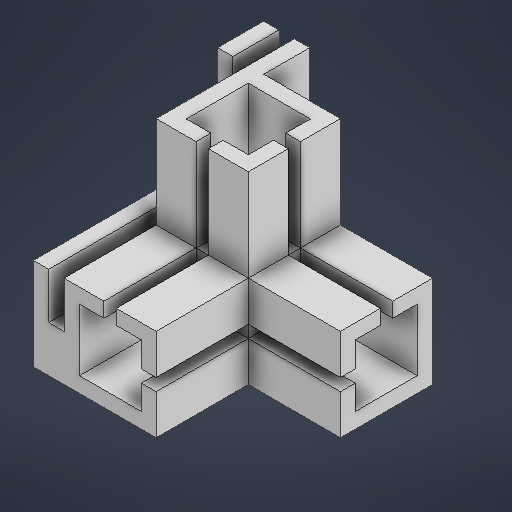
# Autodesk Inventor part: corner connector with rails (front right)
Saved by Autodesk Inventor 2026.2 (Build 302298000, 298)
## iProperties
Created: 2025-11-17
Part Number: corner connector with rails (front right)
Material: Generic
Document SubType Name: Modeling
Designer: dongr
Density: 1 g/cm^3
Appearance: Default
Author: dongr
Autodesk Inventor part; units mm, degrees
ref_plane "YZ Plane" through (0, 0, 0) normal (1, 0, 0) x (0, 1, 0)
ref_plane "XZ Plane" through (0, 0, 0) normal (0, 1, 0) x (-1, 0, 0)
ref_plane "XY Plane" through (0, 0, 0) normal (0, 0, 1) x (1, 0, 0)
sketch "Sketch1" plane through (0, 0, 0) normal (0, 0, 1) x (1, 0, 0)
  line L0 (0, 0) -> (38.1, 0)
  line L1 (38.1, 0) -> (38.1, 38.1)
  line L2 (38.1, 38.1) -> (0, 38.1)
  line L3 (0, 38.1) -> (0, 0)
  dimension "d0" = 38.1
  dimension "d1" = 38.1
  constraints: 8 end point, 2 parallel, 1 horizontal, 1 perpendicular
  measures "d0" distance of L2.end L1.end
  measures "d1" distance of L1.end L0.end
extrude "Extrusion1" add sketch "Sketch1" along normal blind 38.1
sketch "Sketch2" plane through (0, 0, 38.1) normal (0, 0, 1) x (1, 0, 0)
  line L0 (6.35, 6.35) -> (32.004, 6.35)
  line L1 (32.004, 6.35) -> (32.004, 32.004)
  line L2 (32.004, 32.004) -> (6.35, 32.004)
  line L3 (6.35, 32.004) -> (6.35, 6.35)
  line L4 (38.1, 0) -> (38.1, 38.1) projected
  line L5 (0, 0) -> (38.1, 0)
  line L6 (38.1, 0) -> (38.1, 38.1)
  line L7 (38.1, 38.1) -> (0, 38.1)
  line L8 (0, 38.1) -> (0, 0)
  dimension "d4" = 25.654
  dimension "d5" = 25.654
  constraints: 16 end point, 4 parallel, 2 horizontal, 2 perpendicular
  measures "d4" distance of L2.end L1.end
  measures "d5" distance of L1.end L0.end
extrude "Extrusion2" cut sketch "Sketch2" against normal blind 31.75 contours L3 L2 L1 L0
sketch "Sketch5" plane through (0, 0, 38.1) normal (0, 0, 1) x (1, 0, 0)
  line L0 (6.35, 6.35) -> (6.35, 32.004) projected
  line L1 (6.35, 6.35) -> (32.004, 6.35)
  line L2 (32.004, 6.35) -> (32.004, 32.004)
  line L3 (32.004, 32.004) -> (6.35, 32.004)
  line L4 (6.35, 32.004) -> (6.35, 6.35)
  line L5 (0, 0) -> (38.1, 0) projected
  line L6 (0, 0) -> (38.1, 0)
  line L7 (38.1, 0) -> (38.1, 38.1)
  line L8 (38.1, 38.1) -> (0, 38.1)
  line L9 (0, 38.1) -> (0, 0)
  constraints: 16 end point, 4 parallel, 2 horizontal, 2 perpendicular
extrude "Extrusion4" add sketch "Sketch5" along normal blind 38.1
sketch "Sketch7" plane through (38.1, 0, 0) normal (1, 0, 0) x (0, 0, -1)
  line L0 (0, 0) -> (-76.2, 0) projected
  line L1 (0, 0) -> (-38.1, 0)
  line L2 (-38.1, 0) -> (-38.1, 38.1)
  line L3 (-38.1, 38.1) -> (0, 38.1)
  line L4 (0, 38.1) -> (0, 0)
  line L5 (-76.2, 6.35) -> (-6.35, 6.35) projected
  line L6 (-6.35, 6.35) -> (-32.004, 6.35)
  line L7 (-32.004, 6.35) -> (-32.004, 32.004)
  line L8 (-32.004, 32.004) -> (-6.35, 32.004)
  line L9 (-6.35, 32.004) -> (-6.35, 6.35)
  dimension "d16" = 38.1
  dimension "d17" = 38.1
  dimension "d20" = 25.654
  dimension "d21" = 25.654
  constraints: 16 end point, 4 parallel, 2 horizontal, 2 perpendicular
  measures "d16" distance of L2.end L3.end
  measures "d17" distance of L1.end L2.end
  measures "d20" distance of L7.end L8.end
  measures "d21" distance of L6.end L7.end
extrude "Extrusion6" add sketch "Sketch7" along normal blind 38.1
sketch "Sketch9" plane through (38.1, 6.35, 6.35) normal (1, 0, 0) x (0, 0, -1)
  line L0 (-25.654, 0) -> (-25.654, 25.654) projected
  line L1 (0, 0) -> (0, 25.654) projected
  line L2 (-25.654, 0) -> (0, 0)
  line L3 (0, 0) -> (0, 25.654)
  line L4 (0, 25.654) -> (-25.654, 25.654)
  line L5 (-25.654, 25.654) -> (-25.654, 0)
  point P0 (6.35, -6.35)
  constraints: 8 end point, 2 parallel, 1 horizontal, 1 perpendicular
extrude "Extrusion7" cut sketch "Sketch9" against normal blind 31.75
sketch "Sketch10" plane through (0, 38.1, 76.2) normal (0, 1, 0) x (1, 0, 0)
  line L0 (76.2, 69.85) -> (6.35, 69.85) projected
  line L1 (6.35, 69.85) -> (32.004, 69.85)
  line L2 (32.004, 69.85) -> (32.004, 44.196)
  line L3 (32.004, 44.196) -> (6.35, 44.196)
  line L4 (6.35, 44.196) -> (6.35, 69.85)
  line L5 (38.1, 38.1) -> (38.1, 0) projected
  line L6 (0, 76.2) -> (0, 0) projected
  line L7 (38.1, 38.1) -> (0, 38.1)
  line L8 (0, 38.1) -> (0, 76.2)
  line L9 (0, 76.2) -> (38.1, 76.2)
  line L10 (38.1, 76.2) -> (38.1, 38.1)
  point P0 (0, 38.1)
  dimension "d26" = 25.654
  dimension "d27" = 25.654
  constraints: 16 end point, 4 parallel, 2 horizontal, 2 perpendicular
  measures "d26" distance of L2.end L3.end
  measures "d27" distance of L1.end L2.end
extrude "Extrusion8" add sketch "Sketch10" along normal blind 38.1
sketch "Sketch11" plane through (6.35, 38.1, 6.35) normal (0, 1, 0) x (1, 0, 0)
  line L0 (0, -25.654) -> (25.654, -25.654) projected
  line L1 (25.654, -25.654) -> (0, -25.654)
  line L2 (0, -25.654) -> (0, 0)
  line L3 (0, 0) -> (25.654, 0)
  line L4 (25.654, 0) -> (25.654, -25.654)
  point P0 (-6.35, 6.35)
  constraints: 8 end point, 2 parallel, 1 horizontal, 1 perpendicular
extrude "Extrusion9" cut sketch "Sketch11" against normal blind 6.35
sketch "Sketch12" plane through (0, 76.2, 76.2) normal (0, 1, 0) x (1, 0, 0)
  line L0 (38.1, 55.88) -> (32.004, 55.88)
  line L1 (32.004, 55.88) -> (32.004, 58.42)
  line L2 (32.004, 58.42) -> (38.1, 58.42)
  line L3 (38.1, 58.42) -> (38.1, 55.88)
  point P0 (0, 76.2)
  dimension "d32" = 6.096
  dimension "d33" = 2.54
  constraints: 8 end point, 2 parallel, 1 horizontal, 1 perpendicular
  measures "d32" distance of L1.end L2.end
  measures "d33" distance of L0.end L1.end
extrude "Extrusion10" cut sketch "Sketch12" against normal blind 38.1
sketch "Sketch13" plane through (76.2, 38.1, 38.1) normal (0, 1, 0) x (1, 0, 0)
  line L0 (0, 31.75) -> (0, 6.096) projected
  line L1 (-44.196, 17.78) -> (0, 17.78)
  line L2 (0, 17.78) -> (0, 20.32)
  line L3 (0, 20.32) -> (-44.196, 20.32)
  line L4 (-44.196, 20.32) -> (-44.196, 17.78)
  point P0 (-76.2, 38.1)
  dimension "d36" = 2.54
  constraints: 8 end point, 2 parallel, 1 horizontal, 1 perpendicular, 1 point on line
  measures "d36" distance of L2.end L1.end
extrude "Extrusion11" cut sketch "Sketch13" against normal blind 6.35
sketch "Sketch15" plane through (0, 76.2, 76.2) normal (0, 1, 0) x (1, 0, 0)
  line L0 (17.78, 38.1) -> (20.32, 38.1)
  line L1 (20.32, 38.1) -> (20.32, 44.196)
  line L2 (20.32, 44.196) -> (17.78, 44.196)
  line L3 (17.78, 44.196) -> (17.78, 38.1)
  point P0 (0, 76.2)
  dimension "d39" = 2.54
  dimension "d40" = 6.096
  constraints: 8 end point, 2 parallel, 1 horizontal, 1 perpendicular
  measures "d39" distance of L2.end L1.end
  measures "d40" distance of L1.end L0.end
extrude "Extrusion12" cut sketch "Sketch15" against normal blind 38.1
sketch "Sketch16" plane through (0, 38.1, 76.2) normal (0, 1, 0) x (1, 0, 0)
  line L0 (20.32, 44.196) -> (20.32, 38.1) projected
  line L1 (0, 0) -> (38.1, 0) projected
  line L2 (20.32, 44.196) -> (17.78, 44.196)
  line L3 (17.78, 44.196) -> (17.78, 0)
  line L4 (17.78, 0) -> (20.32, 0)
  line L5 (20.32, 0) -> (20.32, 44.196)
  point P0 (0, 76.2)
  dimension "d43" = 2.54
  constraints: 8 end point, 2 parallel, 1 horizontal, 1 perpendicular, 1 point on line
  measures "d43" distance of L4.end L3.end
extrude "Extrusion13" cut sketch "Sketch16" against normal blind 6.35
sketch "Sketch17" plane through (38.1, 0, 76.2) normal (1, 0, 0) x (0, 0, -1)
  line L0 (38.1, 0) -> (38.1, 38.1) projected
  line L1 (0, 17.78) -> (38.1, 17.78)
  line L2 (38.1, 17.78) -> (38.1, 20.32)
  line L3 (38.1, 20.32) -> (0, 20.32)
  line L4 (0, 20.32) -> (0, 17.78)
  point P0 (76.2, 0)
  dimension "d46" = 2.54
  constraints: 8 end point, 2 parallel, 1 horizontal, 1 perpendicular, 1 point on line
  measures "d46" distance of L2.end L1.end
extrude "Extrusion14" cut sketch "Sketch17" against normal blind 6.35
sketch "Sketch18" plane through (38.1, 0, 38.1) normal (0, 0, 1) x (1, 0, 0)
  line L0 (0, 17.78) -> (38.1, 17.78)
  line L1 (38.1, 17.78) -> (38.1, 20.32)
  line L2 (38.1, 20.32) -> (0, 20.32)
  line L3 (0, 20.32) -> (0, 17.78)
  point P0 (-38.1, 0)
  dimension "d49" = 38.1
  dimension "d50" = 2.54
  constraints: 8 end point, 2 parallel, 1 horizontal, 1 perpendicular
  measures "d49" distance of L2.end L1.end
  measures "d50" distance of L1.end L0.end
extrude "Extrusion15" cut sketch "Sketch18" against normal blind 6.35
sketch "Sketch20" plane through (38.1, 38.1, 38.1) normal (0, 0, 1) x (1, 0, 0)
  line L0 (-17.78, -6.096) -> (-17.78, 38.1) projected
  line L1 (0, 0) -> (-17.78, 0) projected
  line L2 (-17.78, 38.1) -> (-16.51, 38.1)
  line L3 (-16.51, 38.1) -> (-16.51, 0)
  line L4 (-16.51, 0) -> (-17.78, 0)
  line L5 (-17.78, 0) -> (-17.78, 38.1)
  point P0 (-38.1, -38.1)
  dimension "d53" = 1.27
  constraints: 8 end point, 2 parallel, 1 horizontal, 1 perpendicular, 1 point on line
  measures "d53" distance of L3.end L4.end
extrude "Extrusion16" cut sketch "Sketch20" against normal blind 6.35
sketch "Sketch21" plane through (38.1, 38.1, 76.2) normal (0, 1, 0) x (1, 0, 0)
  line L0 (-17.78, 0) -> (-17.78, 44.196) projected
  line L1 (0, 0) -> (-17.78, 0) projected
  line L2 (-17.78, 44.196) -> (-16.51, 44.196)
  line L3 (-16.51, 44.196) -> (-16.51, 0)
  line L4 (-16.51, 0) -> (-17.78, 0)
  line L5 (-17.78, 0) -> (-17.78, 44.196)
  point P0 (-38.1, 76.2)
  dimension "d56" = 1.27
  constraints: 8 end point, 2 parallel, 1 horizontal, 1 perpendicular, 1 point on line
  measures "d56" distance of L3.end L4.end
extrude "Extrusion17" cut sketch "Sketch21" against normal blind 6.35
sketch "Sketch23" plane through (0, 38.1, 38.1) normal (0, 0, 1) x (1, 0, 0)
  line L0 (17.78, 0) -> (17.78, 38.1) projected
  line L1 (17.78, 0) -> (0, 0) projected
  line L2 (17.78, 38.1) -> (16.51, 38.1)
  line L3 (16.51, 38.1) -> (16.51, 0)
  line L4 (16.51, 0) -> (17.78, 0)
  line L5 (17.78, 0) -> (17.78, 38.1)
  point P0 (0, -38.1)
  dimension "d59" = 1.27
  constraints: 8 end point, 2 parallel, 1 horizontal, 1 perpendicular, 1 point on line
  measures "d59" distance of L4.end L3.end
extrude "Extrusion18" cut sketch "Sketch23" against normal blind 6.35
sketch "Sketch24" plane through (0, 38.1, 76.2) normal (0, 1, 0) x (1, 0, 0)
  line L0 (17.78, 44.196) -> (17.78, 0) projected
  line L1 (17.78, 0) -> (0, 0) projected
  line L2 (17.78, 44.196) -> (16.51, 44.196)
  line L3 (16.51, 44.196) -> (16.51, 0)
  line L4 (16.51, 0) -> (17.78, 0)
  line L5 (17.78, 0) -> (17.78, 44.196)
  point P0 (0, 76.2)
  dimension "d62" = 1.27
  constraints: 8 end point, 2 parallel, 1 horizontal, 1 perpendicular, 1 point on line
  measures "d62" distance of L4.end L3.end
extrude "Extrusion19" cut sketch "Sketch24" against normal blind 6.35
sketch "Sketch25" plane through (38.1, 0, 76.2) normal (1, 0, 0) x (0, 0, -1)
  line L0 (38.1, 0) -> (38.1, 17.78) projected
  line L1 (38.1, 17.78) -> (0, 17.78)
  line L2 (0, 17.78) -> (0, 16.51)
  line L3 (0, 16.51) -> (38.1, 16.51)
  line L4 (38.1, 16.51) -> (38.1, 17.78)
  point P0 (76.2, 0)
  dimension "d65" = 38.1
  dimension "d66" = 1.27
  constraints: 8 end point, 2 parallel, 1 horizontal, 1 perpendicular
  measures "d65" distance of L3.end L2.end
  measures "d66" distance of L2.end L1.end
extrude "Extrusion20" cut sketch "Sketch25" against normal blind 6.35
sketch "Sketch26" plane through (38.1, 38.1, 76.2) normal (1, 0, 0) x (0, 0, -1)
  line L0 (0, -17.78) -> (38.1, -17.78) projected
  line L1 (38.1, -17.78) -> (0, -17.78)
  line L2 (0, -17.78) -> (0, -16.51)
  line L3 (0, -16.51) -> (38.1, -16.51)
  line L4 (38.1, -16.51) -> (38.1, -17.78)
  point P0 (76.2, -38.1)
  dimension "d69" = 38.1
  dimension "d70" = 1.27
  constraints: 8 end point, 2 parallel, 1 horizontal, 1 perpendicular
  measures "d69" distance of L2.end L3.end
  measures "d70" distance of L1.end L2.end
extrude "Extrusion21" cut sketch "Sketch26" against normal blind 6.35
sketch "Sketch27" plane through (38.1, 0, 38.1) normal (0, 0, 1) x (1, 0, 0)
  line L0 (0, 21.59) -> (0, 38.1) projected
  line L1 (0, 20.32) -> (38.1, 20.32) projected
  line L2 (0, 21.59) -> (38.1, 21.59)
  line L3 (38.1, 21.59) -> (38.1, 20.32)
  line L4 (38.1, 20.32) -> (0, 20.32)
  line L5 (0, 20.32) -> (0, 21.59)
  line L6 (38.1, 17.78) -> (0, 17.78) projected
  line L7 (0, 17.78) -> (38.1, 17.78)
  line L8 (38.1, 17.78) -> (38.1, 16.51)
  line L9 (38.1, 16.51) -> (0, 16.51)
  line L10 (0, 16.51) -> (0, 17.78)
  point P0 (-38.1, 0)
  dimension "d73" = 38.1
  dimension "d74" = 1.27
  constraints: 16 end point, 4 parallel, 2 horizontal, 2 perpendicular
  measures "d73" distance of L8.end L9.end
  measures "d74" distance of L7.end L8.end
extrude "Extrusion22" cut sketch "Sketch27" against normal blind 6.35
sketch "Sketch28" plane through (38.1, 38.1, 38.1) normal (0, 1, 0) x (1, 0, 0)
  line L0 (0, 20.32) -> (38.1, 20.32) projected
  line L1 (0, 20.32) -> (38.1, 20.32)
  line L2 (38.1, 20.32) -> (38.1, 21.59)
  line L3 (38.1, 21.59) -> (0, 21.59)
  line L4 (0, 21.59) -> (0, 20.32)
  line L5 (-6.096, 17.78) -> (38.1, 17.78) projected
  line L6 (38.1, 17.78) -> (0, 17.78)
  line L7 (0, 17.78) -> (0, 16.51)
  line L8 (0, 16.51) -> (38.1, 16.51)
  line L9 (38.1, 16.51) -> (38.1, 17.78)
  point P0 (-38.1, 38.1)
  point P1 (0, 17.78)
  dimension "d77" = 38.1
  dimension "d78" = 1.27
  dimension "d79" = 38.1
  dimension "d80" = 1.27
  constraints: 16 end point, 4 parallel, 2 horizontal, 2 perpendicular
  measures "d77" distance of L3.end L2.end
  measures "d78" distance of L2.end L1.end
  measures "d79" distance of L8.end L7.end
  measures "d80" distance of L7.end L6.end
extrude "Extrusion23" cut sketch "Sketch28" against normal blind 6.35
sketch "Sketch29" plane through (38.1, 38.1, 0) normal (1, 0, 0) x (0, 0, -1)
  line L0 (-17.78, -6.096) -> (-6.35, -6.096) projected
  line L1 (-6.35, 38.1) -> (-17.78, 38.1) projected
  line L2 (-17.78, -6.096) -> (-16.51, -6.096)
  line L3 (-16.51, -6.096) -> (-16.51, 38.1)
  line L4 (-16.51, 38.1) -> (-17.78, 38.1)
  line L5 (-17.78, 38.1) -> (-17.78, -6.096)
  line L6 (-21.59, 0) -> (-21.59, -6.096) projected
  line L7 (-20.32, 38.1) -> (-20.32, -6.096) projected
  line L8 (-21.59, -6.096) -> (-20.32, -6.096)
  line L9 (-20.32, -6.096) -> (-20.32, 38.1)
  line L10 (-20.32, 38.1) -> (-21.59, 38.1)
  line L11 (-21.59, 38.1) -> (-21.59, -6.096)
  point P0 (0, -38.1)
  point P1 (-20.32, -6.096)
  dimension "d83" = 1.27
  constraints: 16 end point, 4 parallel, 2 horizontal, 2 perpendicular, 1 point on line
  measures "d83" distance of L4.end L3.end
extrude "Extrusion24" cut sketch "Sketch29" against normal blind 6.35
sketch "Sketch30" plane through (76.2, 38.1, 21.59) normal (0, 0, -1) x (-1, 0, 0)
  line L0 (0, 0) -> (38.1, 0) projected
  line L1 (44.196, 38.1) -> (44.196, -6.096) projected
  line L2 (38.1, 0) -> (44.196, 0)
  line L3 (44.196, 0) -> (44.196, -6.096)
  line L4 (44.196, -6.096) -> (38.1, -6.096)
  line L5 (38.1, -6.096) -> (38.1, 0)
  point P0 (76.2, -38.1)
  point P1 (44.196, 0)
  constraints: 8 end point, 2 parallel, 1 horizontal, 1 perpendicular
extrude "Extrusion25" add sketch "Sketch30" along normal blind 5.08
sketch "Sketch31" plane through (21.59, 38.1, 38.1) normal (-1, 0, 0) x (0, 0, 1)
  line L0 (38.1, -6.096) -> (-6.096, -6.096) projected
  line L1 (0, 0) -> (-6.096, 0)
  line L2 (-6.096, 0) -> (-6.096, -6.096)
  line L3 (-6.096, -6.096) -> (0, -6.096)
  line L4 (0, -6.096) -> (0, 0)
  point P0 (-38.1, -38.1)
  constraints: 8 end point, 2 parallel, 1 horizontal, 1 perpendicular
extrude "Extrusion26" add sketch "Sketch31" along normal blind 5.08
sketch "Sketch32" plane through (0, 0, 76.2) normal (-1, 0, 0) x (0, 0, 1)
  line L0 (0, 38.1) -> (0, 0) projected
  line L1 (0, 19.05) -> (-76.2, 19.05)
  line L2 (-76.2, 19.05) -> (-76.2, 0)
  line L3 (-76.2, 0) -> (0, 0)
  line L4 (0, 0) -> (0, 19.05)
  line L5 (-76.2, 0) -> (-56.896, 0)
  line L6 (-56.896, 0) -> (-56.896, 76.2)
  line L7 (-56.896, 76.2) -> (-76.2, 76.2)
  line L8 (-76.2, 76.2) -> (-76.2, 0)
  point P0 (0, 0)
  point P1 (-56.896, 19.05)
  dimension "d90" = 19.304
  dimension "d91" = 76.2
  constraints: 16 end point, 4 parallel, 2 horizontal, 2 perpendicular, 1 midpoint
  measures "d90" distance of L7.end L6.end
  measures "d91" distance of L6.end L5.end
extrude "Extrusion27" add sketch "Sketch32" along normal blind 12.7 contours L0 L3 L6 L1 | L6 L3 L2 L1
sketch "Sketch34" plane through (-12.7, 0, 76.2) normal (-1, 0, 0) x (0, 0, 1)
  line L0 (0, 38.1) -> (0, 19.05) projected
  line L1 (0, 19.05) -> (-76.2, 19.05)
  line L2 (-76.2, 19.05) -> (-76.2, 38.1)
  line L3 (-76.2, 38.1) -> (0, 38.1)
  line L4 (0, 38.1) -> (0, 19.05)
  point P0 (-76.2, 0)
  dimension "d98" = 76.2
  dimension "d99" = 19.05
  constraints: 8 end point, 2 parallel, 1 horizontal, 1 perpendicular
  measures "d98" distance of L2.end L3.end
  measures "d99" distance of L1.end L2.end
extrude "Extrusion29" add sketch "Sketch34" against normal blind 6.35
sketch "Sketch35" plane through (-12.7, 0, 76.2) normal (-1, 0, 0) x (0, 0, 1)
  line L0 (-76.2, 0) -> (-95.25, 0)
  line L1 (-95.25, 0) -> (-95.25, 76.2)
  line L2 (-95.25, 76.2) -> (-76.2, 76.2)
  line L3 (-76.2, 76.2) -> (-76.2, 0)
  dimension "d102" = 19.05
  dimension "d103" = 76.2
  constraints: 8 end point, 2 parallel, 1 horizontal, 1 perpendicular
  measures "d102" distance of L1.end L2.end
  measures "d103" distance of L0.end L1.end
extrude "Extrusion30" add sketch "Sketch35" against normal blind 6.35
sketch "Sketch37" plane through (0, 19.05, 76.2) normal (0, 1, 0) x (1, 0, 0)
  line L0 (0, 76.2) -> (-6.35, 76.2)
  line L1 (-6.35, 76.2) -> (-6.35, 95.25)
  line L2 (-6.35, 95.25) -> (0, 95.25)
  line L3 (0, 95.25) -> (0, 76.2)
  dimension "d106" = 6.35
  dimension "d107" = 19.05
  constraints: 8 end point, 2 parallel, 1 horizontal, 1 perpendicular
  measures "d106" distance of L1.end L2.end
  measures "d107" distance of L0.end L1.end
extrude "Extrusion31" add sketch "Sketch37" against normal blind 19.05
sketch "Sketch38" plane through (38.1, 0, 38.1) normal (0, -1, 0) x (1, 0, 0)
  line L0 (-38.1, -38.1) -> (-31.75, -38.1)
  line L1 (-31.75, -38.1) -> (-31.75, -57.15)
  line L2 (-31.75, -57.15) -> (-38.1, -57.15)
  line L3 (-38.1, -57.15) -> (-38.1, -38.1)
  dimension "d110" = 6.35
  dimension "d111" = 19.05
  constraints: 8 end point, 2 parallel, 1 horizontal, 1 perpendicular
  measures "d110" distance of L1.end L2.end
  measures "d111" distance of L0.end L1.end
extrude "Extrusion32" add sketch "Sketch38" against normal blind 76.2
sketch "Sketch39" plane through (-12.7, 0, 76.2) normal (-1, 0, 0) x (0, 0, 1)
  circle A0 centre (-86.36, 50.8) radius 3.81
  point P0 (-76.2, 0)
  dimension "d114" = 7.62
  constraints: 1 centre point
  measures "d114" diameter of A0
extrude "Extrusion33" cut sketch "Sketch39" against normal through all
body "Solid1"
